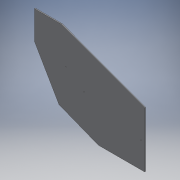
# Autodesk Inventor part: endplate(flap4)
Saved by Autodesk Inventor 2018.2 (Build 222227000, 227)
## iProperties
Created: 2018-02-23
Part Number: endplate(flap4)
Material: 一般
Document SubType Name: Modeling
Designer: ku_sk
Density: 1 g/cm^3
Appearance: 既定
Author: ku_sk
Autodesk Inventor part; units mm, degrees
ref_plane "YZ Plane" through (0, 0, 0) normal (1, 0, 0) x (0, 1, 0)
ref_plane "XZ Plane" through (0, 0, 0) normal (0, 1, 0) x (-1, 0, 0)
ref_plane "XY Plane" through (0, 0, 0) normal (0, 0, 1) x (1, 0, 0)
sketch "スケッチ1" plane through (0, 0, 0) normal (0, 1, 0) x (-1, 0, 0)
  line L0 (-277.5, 277.5) -> (277.5, 277.5)
  line L1 (277.5, 277.5) -> (277.5, -277.5)
  line L2 (277.5, -277.5) -> (-277.5, -277.5)
  line L3 (-277.5, -277.5) -> (-277.5, 277.5)
  line L4 (-277.5, 277.5) -> (277.5, -277.5) construction
  line L5 (277.5, 277.5) -> (-277.5, -277.5) construction
  point P0 (0, 0)
  dimension "d0" = 555
  dimension "d1" = 555
  constraints: 12 end point, 2 midpoint, 2 parallel, 1 horizontal, 1 perpendicular
  measures "d0" distance of L0.start L0.end
  measures "d1" distance of L2.end L0.start
extrude "押し出し1" add sketch "スケッチ1" along normal mid plane 5
sketch "スケッチ3" plane through (0, -2.5, 0) normal (0, -1, 0) x (1, 0, 0)
  circle A0 centre (-62.5, 117.5) radius 2.5
  line L0 (277.5, -277.5) -> (277.5, 277.5) projected
  line L1 (-277.5, -277.5) -> (277.5, -277.5) projected
  circle A1 centre (-162.5, 187.5) radius 2.5
  circle A2 centre (257.5, 42.5) radius 2.5
  point P0 (0, 0)
  dimension "d10" = 5
  dimension "d15" = 5
  dimension "d16" = 320
  dimension "d17" = 20
  dimension "d18" = 5
  dimension "d24" = 75
  dimension "d25" = 320
  dimension "d26" = 420
  dimension "d27" = 145
  constraints: 3 centre point
  measures "d10" diameter of A0
  measures "d15" diameter of A1
  measures "d16" distance from line of L1 A2.centre
  measures "d17" distance from line of L0 A2.centre
  measures "d18" diameter of A2
  measures "d24" vertical distance of A0.centre A2.centre
  measures "d25" horizontal distance of A0.centre A2.centre
  measures "d26" horizontal distance of A1.centre A2.centre
  measures "d27" vertical distance of A2.centre A1.centre
extrude "押し出し4" cut sketch "スケッチ3" against normal through all
sketch "スケッチ5" plane through (0, -2.5, 0) normal (0, -1, 0) x (1, 0, 0)
  line L0 (277.5, 250) -> (-277.5, 250)
  line L1 (-250, 277.5) -> (-250, -277.5) construction
  line L2 (-277.5, -250) -> (277.5, -250)
  line L3 (250, -277.5) -> (250, 277.5) construction
  line L4 (-277.5, 277.5) -> (277.5, 277.5)
  line L5 (-150, 277.5) -> (277.5, 120)
  line L6 (277.5, 277.5) -> (277.5, -277.5)
  line L7 (-277.5, -277.5) -> (-277.5, 277.5)
  line L8 (-277.5, 120) -> (-150.482941, -100)
  line L9 (-150.482941, -100) -> (277.5, -100)
  line L10 (277.5, -277.5) -> (277.5, 277.5)
  point P0 (0, 0)
  dimension "d32" = 100
  dimension "d33" = 130
  dimension "d34" = 350
  dimension "d35" = 60
  dimension "d46" = 220
  constraints: 6 end point, 4 point on line, 1 horizontal, 1 vertical alignment
  measures "d32" distance from line of L5.start L1
  measures "d33" distance from line of L0 L8.start
  measures "d34" distance between parallel lines of L0 L9
  measures "d35" angle of L9 L8
  measures "d46" distance of L9.end L5.end
sketch "スケッチ5 outline for 押し出し5" plane through (0, -2.5, 0) normal (0, -1, 0) x (1, 0, 0)
  line L0 (277.5, 120) -> (277.5, 277.5)
  line L1 (-150, 277.5) -> (277.5, 120)
  line L2 (277.5, 277.5) -> (-150, 277.5)
  line L3 (-277.5, 120) -> (-277.5, -277.5)
  line L4 (-150.482941, -100) -> (-277.5, 120)
  line L5 (277.5, -100) -> (-150.482941, -100)
  line L6 (277.5, -277.5) -> (277.5, -100)
  line L7 (-277.5, -277.5) -> (277.5, -277.5)
extrude "押し出し5" cut sketch "スケッチ5 outline for 押し出し5" against normal through all
chamfer "面取り2" distance 170 distance2 100 1 edges at (-150.4829, 0, -100) measured on face at (134.839, -0.8333, -100)
sketch "スケッチ6" plane through (0, 2.5, 0) normal (0, 1, 0) x (1, 0, 0)
  line L0 (277.5, -120) -> (-150, -277.5)
  line L1 (277.5, -120) -> (277.5, -238.748566)
  line L2 (277.5, -238.748566) -> (-133.265714, -390.083302)
  line L3 (-133.265714, -390.083302) -> (-342.5, -390.083302)
  line L4 (-342.5, -390.083302) -> (-342.5, -232.583302)
  line L5 (-277.5, -277.5) -> (-277.5, -120)
  line L6 (-342.5, -232.583302) -> (-277.5, -120)
  line L7 (-200.482941, 13.39746) -> (-277.5, -120)
  line L8 (-277.5, -277.5) -> (-150, -277.5)
  point P0 (0, 0)
  dimension "d47" = 157.5
  dimension "d55" = 620
  constraints: 10 end point, 2 perpendicular, 1 collinear, 1 parallel, 1 vertical
  measures "d47" distance of L3.end L4.end
  measures "d55" distance between parallel lines of L1 L4
extrude "押し出し6" add sketch "スケッチ6" against normal blind 5
sketch "スケッチ7" plane through (0, 2.5, 0) normal (0, 1, 0) x (1, 0, 0)
  circle A0 centre (-242.5, -283) radius 2.5
  line L0 (277.5, -238.748566) -> (277.5, 100)
  line L1 (277.5, 100) -> (19.517059, 100)
  point P0 (0, 0)
  dimension "d50" = 5
  dimension "d51" = 520
  dimension "d52" = 383
  constraints: 1 centre point
  measures "d50" diameter of A0
  measures "d51" distance from line of L0 A0.centre
  measures "d52" distance from line of L1 A0.centre
extrude "押し出し7" cut sketch "スケッチ7" against normal through all
